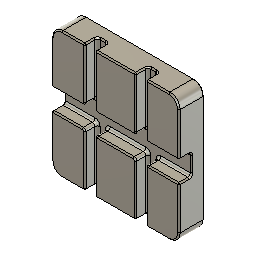
P1S_foot_base (Autodesk Fusion 360 design; units mm, degrees)
Autodesk Fusion 360 part; units mm, degrees
sketch "スケッチ1" plane through (0, 0, 0) normal (0, 0, 1) x (1, 0, 0)
  line L0 (-25, 25) -> (25, 25)
  line L1 (25, 25) -> (25, -25)
  line L2 (25, -25) -> (-25, -25)
  line L3 (-25, -25) -> (-25, 25)
  line L4 (0, 1.75) -> (0, 22.5)
  line L5 (1.75, 0) -> (22.5, 0)
  line L6 (-10, -25) -> (-10, 25)
  line L7 (10, -25) -> (10, 25)
  line L8 (-12, 25) -> (-12, -25)
  line L9 (-8, -25) -> (-8, 25)
  line L10 (8, 25) -> (8, -25)
  line L11 (12, -25) -> (12, 25)
  line L12 (-25, 4) -> (25, 4)
  line L13 (25, -4) -> (-25, -4)
  line L14 (30, -25) -> (30, 25)
  line L15 (-30, -25) -> (-30, 25)
  line L16 (32, -25) -> (32, 25)
  line L17 (28, 25) -> (28, -25)
  line L18 (-28, -25) -> (-28, 25)
  line L19 (-32, 25) -> (-32, -25)
  dimension "d1" = 50
  dimension "d2" = 50
  dimension "d5" = 20
  dimension "d8" = 4
  dimension "d9" = 4
  dimension "d10" = 8
  dimension "d18" = 20
  dimension "d19" = 20
  dimension "d20" = 4
  dimension "d21" = 4
  constraint horizontal L0
  constraint vertical L1
  constraint horizontal L2
  constraint vertical L3
  constraint symmetric L1 L3 L4
  constraint symmetric L0 L2 L5
  constraint coincident L2 L6.start
  constraint coincident L0 L6.end
  constraint perpendicular L0 L6
  constraint coincident L2 L7.start
  constraint coincident L0 L7.end
  constraint vertical L7
  constraint symmetric L4 L6 L7
  constraint coincident L0 L8.start
  constraint coincident L2 L8.end
  constraint perpendicular L2 L8
  constraint coincident L2 L9.start
  constraint coincident L0 L9.end
  constraint perpendicular L0 L9
  constraint coincident L0 L10.start
  constraint coincident L2 L10.end
  constraint perpendicular L2 L10
  constraint coincident L2 L11.start
  constraint coincident L0 L11.end
  constraint perpendicular L0 L11
  constraint symmetric L6 L8 L9
  constraint symmetric L7 L10 L11
  constraint coincident L3 L12.start
  constraint coincident L1 L12.end
  constraint perpendicular L1 L12
  constraint coincident L1 L13.start
  constraint coincident L3 L13.end
  constraint perpendicular L3 L13
  constraint symmetric L5 L12 L13
  constraint coincident L2 L14.start
  constraint coincident L0 L14.end
  constraint perpendicular L0 L14
  constraint coincident L2 L15.start
  constraint coincident L0 L15.end
  constraint perpendicular L0 L15
  constraint coincident L2 L16.start
  constraint coincident L0 L16.end
  constraint coincident L0 L17.start
  constraint coincident L2 L17.end
  constraint perpendicular L2 L17
  constraint coincident L2 L18.start
  constraint coincident L0 L18.end
  constraint perpendicular L0 L18
  constraint coincident L0 L19.start
  constraint coincident L2 L19.end
  constraint perpendicular L2 L19
  constraint symmetric L15 L18 L19
  measures "d1" distance of L0.start L0.end
  measures "d2" distance of L0.start L2.end
  measures "d5" distance of L6 L7
  measures "d8" distance of L8 L9
  measures "d9" distance of L10 L11
  measures "d10" distance of L12 L13
  measures "d18" distance of L6.start L15.start
  measures "d19" distance of L7.start L14.start
  measures "d20" distance of L16 L17
  measures "d21" distance of L18 L19
extrude "押し出し1" add sketch "スケッチ1" along normal blind 5
extrude "押し出し2" add sketch "スケッチ1" against normal blind 5
extrude "押し出し3" cut sketch "スケッチ1" along normal through all contours L0 L6 L8 L12 | L3 L8 L12 L13 | L0 L6 L9 L12 | L6 L8 L12 L13 | L6 L9 L12 L13 | L2 L6 L8 L13 | L0 L7 L10 L12 | L9 L10 L12 L13 | L2 L6 L9 L13 | L0 L7 L11 L12 | L5 L7 L10 L12 | L5 L7 L11 L12 | L5 L7 L10 L13 | L2 L7 L10 L13 | L1 L11 L12 L13 | L5 L7 L11 L13 | L2 L7 L11 L13
fillet "フィレット1" radius 4 4 edges at (-25, 25, 0) (25, 25, 0) (25, -25, 0) (-25, -25, 0)
fillet "フィレット2" radius 1 22 edges at (8, 14.5, 0) (12, 14.5, 0) (18.5, 4, 0) (0, 4, 0) (-18.5, 4, 0) (-8, 14.5, 0) (-8, -14.5, 0) (12, -14.5, 0) (-12, -14.5, 0) (-18.5, -4, 0) (8, -14.5, 0) (0, -4, 0) (18.5, -4, 0) (-12, 14.5, 0) (8, -4, 2.5) (-12, -4, 2.5) (-12, 4, 2.5) (8, 4, 2.5) (12, 4, 2.5) (12, -4, 2.5) (-8, 4, 2.5) (-8, -4, 2.5)
sketch "スケッチ2" plane through (0, 0, -5) normal (0, 0, -1) x (-1, 0, 0)
  arc A0 (21, -25) -> (25, -21) centre (21, -21) ccw
  line L0 (25, -21) -> (25, 21)
  arc A1 (25, 21) -> (21, 25) centre (21, 21) ccw
  line L1 (21, 25) -> (-21, 25)
  arc A2 (-21, 25) -> (-25, 21) centre (-21, 21) ccw
  line L2 (-25, 21) -> (-25, -21)
  arc A3 (-25, -21) -> (-21, -25) centre (-21, -21) ccw
  line L3 (-21, -25) -> (21, -25)
sketch "スケッチ3" plane through (0, 0, -5) normal (0, 0, -1) x (-1, 0, 0)
  circle A0 centre (0, 0) radius 21
  arc A1 (21, -25) -> (25, -21) centre (21, -21) ccw
  line L0 (25, -21) -> (25, 21)
  arc A2 (25, 21) -> (21, 25) centre (21, 21) ccw
  line L1 (21, 25) -> (-21, 25)
  arc A3 (-21, 25) -> (-25, 21) centre (-21, 21) ccw
  line L2 (-25, 21) -> (-25, -21)
  arc A4 (-25, -21) -> (-21, -25) centre (-21, -21) ccw
  line L3 (-21, -25) -> (21, -25)
  dimension "d22" = 42
  constraint coincident A0.centre origin
  measures "d22" diameter of A0
extrude "押し出し4" cut sketch "スケッチ3" against normal blind 4 contours A0
chamfer "面取り1" distance 0.5 angle 45 15 faces at (-20.4647, -20.0945, -5) (-17.9966, 25, 0.2859) (23.4726, 24.1442, 1.6667) (25, 15.3299, 0.2859) (21.1903, -24.9955, -1.6667) (17.9966, -25, 0.2859) (-21.1903, -24.9955, -1.6667) (-25, 15.3299, 0.2859) (-24.9955, 21.1903, -1.6667) (-2.6667, 18.3333, 5) (-16.3333, 17, 5) (-16.3333, -17, 5) (-2.6667, -11.6667, 5) (16.3333, -17, 5) (16.3333, 17, 5)
fillet "フィレット3" radius 0.5 1 edges at (19.5789, 7.5939, -1)
equation "d20 = d9"
equation "d21 = d20"
